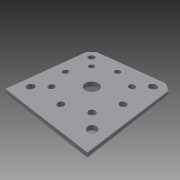
# Autodesk Inventor part: MOTOR001
Saved by Autodesk Inventor 2015 SP1 (Build 190203100, 203)
## iProperties
Created: 2015-06-14
Part Number: MOTOR001
Material: Generic
Document SubType Name: Modeling
Designer: rhornbak
Density: 1 g/cm^3
Appearance: Default
Author: rhornbak
Autodesk Inventor part; units mm, degrees
ref_plane "YZ Plane" through (0, 0, 0) normal (1, 0, 0) x (0, 1, 0)
ref_plane "XZ Plane" through (0, 0, 0) normal (0, 1, 0) x (-1, 0, 0)
ref_plane "XY Plane" through (0, 0, 0) normal (0, 0, 1) x (1, 0, 0)
sketch "Sketch1" plane through (0, 0, 0) normal (0, 0, 1) x (1, 0, 0)
  line L0 (26.75, 31.75) -> (-26.75, 31.75)
  line L1 (-31.75, 26.75) -> (-31.75, -34.45)
  line L2 (-31.75, -34.45) -> (31.75, -34.45)
  line L3 (31.75, -34.45) -> (31.75, 26.75)
  circle A0 centre (0, 0) radius 5
  circle A1 centre (15.5, 15.5) radius 2.25
  circle A2 centre (-15.5, 15.5) radius 2.25
  circle A3 centre (-15.5, -15.5) radius 2.25
  circle A4 centre (15.5, -15.5) radius 2.25
  line L4 (-15.5, -15.5) -> (15.5, -15.5) construction
  line L5 (15.5, -15.5) -> (15.5, 15.5) construction
  line L6 (15.5, 15.5) -> (-15.5, 15.5) construction
  line L7 (-15.5, 15.5) -> (-15.5, -15.5) construction
  line L8 (0, 2.2207) -> (0, -2.8787) construction
  line L9 (-1.8221, 0) -> (3.1794, 0) construction
  circle A5 centre (0, 21.9203) radius 2.25
  circle A6 centre (0, -21.9203) radius 2.25
  circle A7 centre (-21.9203, 0) radius 2.25
  circle A8 centre (21.9203, 0) radius 2.25
  line L10 (0, 21.9203) -> (-21.9203, 0) construction
  line L11 (-21.9203, 0) -> (0, -21.9203) construction
  line L12 (0, -21.9203) -> (21.9203, 0) construction
  line L13 (21.9203, 0) -> (0, 21.9203) construction
  line L14 (-23.57, 23.57) -> (23.57, 23.57) construction
  line L15 (23.57, 23.57) -> (23.57, -23.57) construction
  line L16 (23.57, -23.57) -> (-23.57, -23.57) construction
  line L17 (-23.57, -23.57) -> (-23.57, 23.57) construction
  circle A9 centre (-23.57, 23.57) radius 2.75
  circle A10 centre (-23.57, -23.57) radius 2.75
  circle A11 centre (23.57, -23.57) radius 2.75
  circle A12 centre (23.57, 23.57) radius 2.75
  line L18 (-23.6, 28.2) -> (23.6, 28.2) construction
  line L19 (28.2, 23.6) -> (28.2, -23.6) construction
  line L20 (23.6, -28.2) -> (-23.6, -28.2) construction
  line L21 (-28.2, -23.6) -> (-28.2, 23.6) construction
  arc A13 (-23.6, 28.2) -> (-28.2, 23.6) centre (-23.6, 23.6) ccw construction
  arc A14 (-28.2, -23.6) -> (-23.6, -28.2) centre (-23.6, -23.6) ccw construction
  arc A15 (23.6, -28.2) -> (28.2, -23.6) centre (23.6, -23.6) ccw construction
  arc A16 (28.2, 23.6) -> (23.6, 28.2) centre (23.6, 23.6) ccw construction
  line L22 (-31.75, 26.75) -> (-26.75, 31.75)
  line L23 (26.75, 31.75) -> (31.75, 26.75)
  line L24 (-15.5, 21) -> (15.5, 21) construction
  line L25 (21, 15.5) -> (21, -15.5) construction
  line L26 (15.5, -21) -> (-15.5, -21) construction
  line L27 (-21, -15.5) -> (-21, 15.5) construction
  line L28 (-21, 15.5) -> (-15.5, 21) construction
  line L29 (15.5, 21) -> (21, 15.5) construction
  line L30 (21, -15.5) -> (15.5, -21) construction
  line L31 (-15.5, -21) -> (-21, -15.5) construction
  point P0 (-31.75, 31.75)
  point P1 (-31.75, 31.75)
  point P2 (31.75, 31.75)
  point P3 (28.2, -28.2)
  point P4 (-28.2, -28.2)
  point P5 (-31.75, 31.75)
  point P6 (31.75, 31.75)
  point P7 (-21, 21)
  point P8 (21, -21)
  point P9 (21, 21)
  point P10 (-21, -21)
  dimension "MotorPlateWidth" = 63.5
  dimension "MotorPlateHeight" = 66.2
  dimension "d5" = 31.75
  dimension "ShaftHole" = 10
  dimension "d10" = 4.5
  dimension "NEMA17HoleSpacing" = 31
  dimension "NEMA23HoleSpacing" = 47.14
  dimension "NEMA23MountingHole" = 5.5
  dimension "NEMA23Motor" = 56.4
  dimension "d35" = 4.6
  dimension "CornerChamfer" = 5
  dimension "d37" = 5
  dimension "d38" = 5
  dimension "d39" = 5
  dimension "NEMA17Motor" = 42
  dimension "NEMA17CornerChamfer" = 5.5
  dimension "d42" = 5.5
  dimension "d43" = 5.5
  dimension "d44" = 5.5
  dimension "d45" = 5.5
  dimension "d46" = 5.5
  dimension "d47" = 5.5
  dimension "d48" = 5.5
  constraints: 64 end point, 24 point on line, 17 centre point, 14 coincident, 13 equal radius, 12 parallel, 8 point on circle, 8 tangent, 6 equal length, 6 horizontal, 6 perpendicular, 2 symmetric about line, 1 vertical, 9 other
  measures "MotorPlateWidth" distance of L2.end L1.end
  measures "MotorPlateHeight" distance of L1.end point (-31.75, 31.75)
  measures "d5" distance from line of L0 point (0, 0)
  measures "ShaftHole" diameter of A0
  measures "d10" diameter of A2
  measures "NEMA17HoleSpacing" distance of L6.end L5.end
  measures "NEMA23HoleSpacing" distance of L15.end L16.end
  measures "NEMA23MountingHole" diameter of A9
  measures "NEMA23Motor" distance of point (28.2, -28.2) point (-28.2, -28.2)
  measures "d35" radius of A13
  measures "CornerChamfer" distance of L1.start point (-31.75, 31.75)
  measures "d37" distance of L0.end point (-31.75, 31.75)
  measures "d38" distance of L0.start point (31.75, 31.75)
  measures "d39" distance of L3.end point (31.75, 31.75)
  measures "NEMA17Motor" distance of point (21, -21) point (-21, -21)
  measures "NEMA17CornerChamfer" distance of L27.end point (-21, 21)
  measures "d42" distance of L24.start point (-21, 21)
  measures "d43" distance of L24.end point (21, 21)
  measures "d44" distance of L25.start point (21, 21)
  measures "d45" distance of L25.end point (21, -21)
  measures "d46" distance of L26.start point (21, -21)
  measures "d47" distance of L26.end point (-21, -21)
  measures "d48" distance of L27.start point (-21, -21)
extrude "Extrusion2" add sketch "Sketch1" along normal mid plane 3.125
fillet "Fillet2" radius 0.5 14 edges at (-31.75, 26.75, 0) (-29.25, 29.25, 1.5625) (-26.75, 31.75, 0) (-29.25, 29.25, -1.5625) (0, 31.75, 1.5625) (26.75, 31.75, 0) (0, 31.75, -1.5625) (29.25, 29.25, 1.5625) (31.75, 26.75, 0) (29.25, 29.25, -1.5625) (-31.75, -3.85, 1.5625) (-31.75, -3.85, -1.5625) (31.75, -3.85, 1.5625) (31.75, -3.85, -1.5625)
equation "\"d5\" = 0.5 * MotorPlateWidth"
equation "\"d10\" = NEMA17MountingHole"
equation "\"d37\" = CornerChamfer"
equation "\"d38\" = CornerChamfer"
equation "\"d39\" = CornerChamfer"
equation "\"d42\" = NEMA17CornerChamfer"
equation "\"d43\" = NEMA17CornerChamfer"
equation "\"d44\" = NEMA17CornerChamfer"
equation "\"d45\" = NEMA17CornerChamfer"
equation "\"d46\" = NEMA17CornerChamfer"
equation "\"d47\" = NEMA17CornerChamfer"
equation "\"d48\" = NEMA17CornerChamfer"
equation "\"NEMA17MountingHole\" = 4.5"
body "Solid2"
